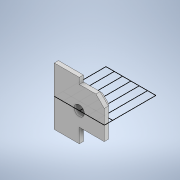
# Autodesk Inventor part: power and ground splitter holders top lid
Saved by Autodesk Inventor 2022 (Build 260153000, 153)
## iProperties
Created: 2022-04-13
Part Number: power and ground splitter holders top lid
Material: Generic
Document SubType Name: Modeling
Designer: a-dubs
Density: 1 g/cm^3
Appearance: Default
Author: a-dubs
Autodesk Inventor part; units mm, degrees
ref_plane "YZ Plane" through (0, 0, 0) normal (1, 0, 0) x (0, 1, 0)
ref_plane "XZ Plane" through (0, 0, 0) normal (0, 1, 0) x (-1, 0, 0)
ref_plane "XY Plane" through (0, 0, 0) normal (0, 0, 1) x (1, 0, 0)
sketch "Sketch1" plane through (0, 0, 0) normal (0, 1, 0) x (-1, 0, 0)
  line L0 (0, 0) -> (-2.6, 0)
  line L1 (-2.6, 0) -> (-2.6, -13.5)
  line L2 (-2.6, 0) -> (-3.6568, 0)
  line L3 (-2.6, -13.5) -> (0, -13.5)
  line L4 (0, -13.5) -> (0, 0)
  line L5 (0, 0) -> (0, 2.6)
  line L6 (0, 2.6) -> (-2.6, 2.6)
  line L7 (-2.6, 2.6) -> (-2.6, 0)
  line L8 (-2.6, 0) -> (-5.2, 0)
  line L9 (-5.2, 0) -> (-5.2, 2.6)
  line L10 (-5.2, 2.6) -> (-2.6, 2.6)
  line L11 (0, 0) -> (2.6, 0)
  line L12 (2.6, 0) -> (2.6, 2.6)
  line L13 (2.6, 2.6) -> (0, 2.6)
  line L14 (2.6, 0) -> (2.6, -13.5)
  line L15 (2.6, -13.5) -> (0, -13.5)
  line L16 (-2.6, -13.5) -> (-5.2, -13.5)
  line L17 (-5.2, -13.5) -> (-5.2, 0)
  line L18 (-10.4, 0) -> (-7.8, 0)
  line L19 (-7.8, 0) -> (-7.8, -13.5)
  line L20 (-7.8, 0) -> (-6.7432, 0)
  line L21 (-7.8, -13.5) -> (-10.4, -13.5)
  line L22 (-10.4, -13.5) -> (-10.4, 0)
  line L23 (-10.4, 0) -> (-10.4, 2.6)
  line L24 (-10.4, 2.6) -> (-7.8, 2.6)
  line L25 (-7.8, 2.6) -> (-7.8, 0)
  line L26 (-7.8, 0) -> (-5.2, 0)
  line L27 (-5.2, 2.6) -> (-7.8, 2.6)
  line L28 (-10.4, 0) -> (-13, 0)
  line L29 (-13, 0) -> (-13, 2.6)
  line L30 (-13, 2.6) -> (-10.4, 2.6)
  line L31 (-13, 0) -> (-13, -13.5)
  line L32 (-13, -13.5) -> (-10.4, -13.5)
  line L33 (-7.8, -13.5) -> (-5.2, -13.5)
  dimension "d0" = 2.6
  dimension "d1" = 13.5
  dimension "d2" = 2.6
  dimension "d3" = 2.6
  dimension "d6" = 2.6
  constraints: 68 end point, 10 perpendicular, 10 symmetric about line, 5 horizontal, 4 point on line, 1 vertical
  measures "d0" distance of L0.start L0.end
  measures "d1" distance of L0.end L1.end
  measures "d2" distance of L0.start L5.end
  measures "d3" distance of L0.end L8.end
  measures "d6" distance of L0.start L11.end
extrude "Extrusion1" add sketch "Sketch1" along normal mid plane 18 contours L0 L7 L6 L5 | L5 L13 L12 L11 | L2 L8 L9 L10 L7
extrude "Extrusion2" add sketch "Sketch1" along normal mid plane 9 contours L26 L20 L25 L27 L9 | L25 L18 L23 L24 | L23 L28 L29 L30
sketch "Sketch3" plane through (5.2, 9, 0) normal (0, 0, -1) x (-1, 0, 0)
  line L0 (7.8, -18) -> (7.8, 0) projected
  line L1 (7.8, -9) -> (0, -9)
  circle A0 centre (0, -9) radius 1.6
  point P0 (5.2, -9)
  dimension "d12" = 7.8
  dimension "d13" = 3.2
  constraints: 2 end point, 1 centre point, 1 coincident, 1 horizontal, 1 midpoint
  measures "d12" distance of L1.start L1.end
  measures "d13" diameter of A0
extrude "Extrusion3" cut sketch "Sketch3" against normal blind 9
extrude "Extrusion4" add sketch "Sketch1" along normal blind 2.6 from surface at 4.5 contours L26 L20 L25 L27 L9 | L25 L18 L23 L24 | L23 L28 L29 L30
chamfer "Chamfer3" distance 2.6 angle 45 1 edges at (13, 7.1, 1.3)
chamfer "Chamfer4" distance 1.3 angle 45 9 edges at (-2.6, 0, 0) (1.3, -9, 0) (9.1, -4.5, 0) (5.2, -6.75, 0) (1.3, 9, 0) (13, 0, 0) (11.7, 5.8, 0) (7.8, 7.1, 0) (5.2, 8.05, 0)
body "Solid1"
